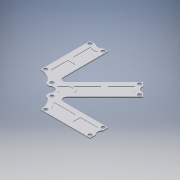
# Autodesk Inventor part: SolarFolds_Sketch
Saved by Autodesk Inventor 2016 (Build 200138000, 138)
## iProperties
Created: 2015-03-28
Part Number: SolarFolds_Sketch
Material: Generic
Document SubType Name: Modeling
Designer: Erin
Density: 1 g/cm^3
Appearance: Default
Author: Erin
Autodesk Inventor part; units mm, degrees
ref_plane "YZ Plane" through (0, 0, 0) normal (1, 0, 0) x (0, 1, 0)
ref_plane "XZ Plane" through (0, 0, 0) normal (0, 1, 0) x (-1, 0, 0)
sketch "Sketch1" plane through (0, 0, 0) normal (0, 0, 1) x (1, 0, 0)
  line L0 (-41.5, 58) -> (41.5, 58)
  line L1 (41.5, 58) -> (41.5, 158)
  line L2 (41.5, 158) -> (-41.5, 158)
  line L3 (-41.5, 158) -> (-41.5, 58)
  line L4 (58, 41.5) -> (158, 41.5)
  line L5 (158, 41.5) -> (158, -41.5)
  line L6 (158, -41.5) -> (58, -41.5)
  line L7 (58, -41.5) -> (58, 41.5)
  line L8 (-131.1952, 0) -> (204.4844, 0) construction
  line L9 (-48, 48) -> (48, 48)
  line L10 (48, 48) -> (48, -48)
  line L11 (48, -48) -> (-48, -48)
  line L12 (-48, -48) -> (-48, 48)
  line L13 (0, 180.9439) -> (0, -136.3054) construction
  point P0 (0, 0)
  point P1 (-48, 0)
  point P2 (0, 48)
  point P3 (0, 58)
  point P4 (58, 0)
  dimension "d0" = 83
  dimension "d1" = 100
  dimension "d2" = 100
  dimension "d3" = 83
  dimension "d5" = 96
  dimension "d6" = 96
  dimension "d7" = 10
  dimension "d8" = 10
  constraints: 28 end point, 7 parallel, 4 horizontal, 4 midpoint, 4 perpendicular, 2 horizontal alignment, 2 vertical alignment, 1 vertical
  measures "d0" distance of L2.end L1.end
  measures "d1" distance of L1.end L0.end
  measures "d2" distance of L5.end L6.end
  measures "d3" distance of L4.end L5.end
  measures "d5" distance of L9.start L9.end
  measures "d6" distance of L11.end L9.start
  measures "d7" distance between parallel lines of L9 L0
  measures "d8" distance between parallel lines of L7 L10
sketch "Sketch2" plane through (0, 0, 0) normal (0, 0, 1) x (1, 0, 0)
  line L0 (41.5, 158) -> (-41.5, 158) projected
  line L1 (41.5, 58) -> (41.5, 158) projected
  line L2 (-48, 48) -> (48, 48) projected
  line L3 (48, 48) -> (48, -48) projected
  line L4 (58, -41.5) -> (58, 41.5) projected
  line L5 (58, 41.5) -> (158, 41.5) projected
  line L6 (-41.5, 58) -> (41.5, 58) projected
  line L7 (158, 41.5) -> (158, -41.5) projected
  line L8 (48, 48) -> (136.7868, 136.7868) construction
  line L9 (35.5, 78) -> (57.5, 78)
  line L10 (57.5, 78) -> (57.5, 138)
  line L11 (57.5, 138) -> (35.5, 138)
  line L12 (35.5, 138) -> (35.5, 78)
  line L13 (41.5, 108) -> (-41.5, 108) construction
  line L14 (108, 41.5) -> (108, -41.5) construction
  line L15 (41.5, 158) -> (220.1006, 158) construction
  line L16 (158, 41.5) -> (158, 206.0131) construction
  line L17 (115.5736, 158) -> (158, 115.5736) construction
  line L18 (41.5, 138) -> (41.5, 78) construction
  line L19 (51.5, 138) -> (51.5, 78) construction
  line L20 (46.5, 138) -> (46.5, 78) construction
  line L21 (51.5, 158) -> (51.5, 70.6421)
  line L22 (60.0355, 67.1066) -> (133.2513, 140.3223)
  arc A0 (51.5, 158) -> (133.2513, 140.3223) centre (109.2071, 226.9991) ccw
  line L23 (68.9045, 84.4609) -> (84.4609, 68.9045)
  line L24 (84.4609, 68.9045) -> (126.8873, 111.331)
  line L25 (126.8873, 111.331) -> (111.331, 126.8873)
  line L26 (111.331, 126.8873) -> (68.9045, 84.4609)
  line L27 (80.2183, 73.1472) -> (122.6447, 115.5736) construction
  line L28 (105.6741, 90.1177) -> (90.1177, 105.6741) construction
  line L29 (73.1472, 80.2183) -> (115.5736, 122.6447) construction
  line L30 (76.6827, 76.6827) -> (119.1091, 119.1091) construction
  circle A1 centre (73.1472, 84.4609) radius 2.25
  circle A2 centre (111.331, 122.6447) radius 2.25
  circle A3 centre (84.4609, 73.1472) radius 2.25
  circle A4 centre (122.6447, 111.331) radius 2.25
  circle A5 centre (38.5, 135) radius 2.25
  circle A6 centre (38.5, 81) radius 2.25
  circle A7 centre (54.5, 135) radius 2.25
  circle A8 centre (54.5, 81) radius 2.25
  arc A9 (51.5, 70.6421) -> (60.0355, 67.1066) centre (56.5, 70.6421) ccw
  point P0 (0, 0)
  point P1 (158, 158)
  dimension "d23" = 30
  dimension "d25" = 45
  dimension "d30" = 10
  dimension "d37" = 10
  dimension "d38" = 60
  dimension "d39" = 4.5
  dimension "d40" = 3
  dimension "d42" = 4.5
  dimension "d43" = 3
  dimension "d46" = 60
  dimension "d47" = 30
  dimension "d48" = 4.5
  dimension "d49" = 3
  dimension "d50" = 3
  dimension "d51" = 4.5
  dimension "d52" = 3
  dimension "d53" = 3
  dimension "d54" = 5
  dimension "d55" = 25
  dimension "d57" = 3
  dimension "d58" = 3
  dimension "d59" = 3
  dimension "d60" = 3
  constraints: 46 end point, 15 perpendicular, 14 point on line, 10 centre point, 9 midpoint, 5 collinear, 4 point on circle, 4 symmetric about line, 3 parallel, 2 tangent, 1 horizontal, 4 other
  measures "d23" distance from line of point (158, 158) L17
  measures "d25" angle of L16 L17
  measures "d30" distance between parallel lines of L18 L19
  measures "d37" distance between parallel lines of L27 L29
  measures "d38" distance of L23.end L24.end
  measures "d39" diameter of A1
  measures "d40" distance from line of A1.centre L26
  measures "d42" diameter of A2
  measures "d43" distance from line of A2.centre L26
  measures "d46" distance of L9.end L10.end
  measures "d47" distance between parallel lines of L13 L11
  measures "d48" diameter of A5
  measures "d49" distance from line of A5.centre L11
  measures "d50" distance from line of A5.centre L12
  measures "d51" diameter of A6
  measures "d52" distance from line of A6.centre L9
  measures "d53" distance from line of A6.centre L12
  measures "d54" radius of A9
  measures "d55" distance between parallel lines of L17 L25
  measures "d57" distance from line of A5.centre L1
  measures "d58" distance from line of A7.centre L21
  measures "d59" distance from line of A4.centre L27
  measures "d60" distance from line of A2.centre L22
sketch "Sketch6" plane through (0, 0, 0) normal (0, 0, 1) x (1, 0, 0)
  line L0 (57.5, 138) -> (35.5, 138) projected
  line L1 (35.5, 138) -> (35.5, 78) projected
  line L2 (35.5, 78) -> (57.5, 78) projected
  circle A0 centre (38.5, 81) radius 2.25 projected
  circle A1 centre (38.5, 135) radius 2.25 projected
  circle A2 centre (54.5, 135) radius 2.25 projected
  line L3 (111.331, 126.8873) -> (68.9045, 84.4609) projected
  circle A3 centre (111.331, 122.6447) radius 2.25 projected
  line L4 (126.8873, 111.331) -> (111.331, 126.8873) projected
  line L5 (84.4609, 68.9045) -> (126.8873, 111.331) projected
  line L6 (68.9045, 84.4609) -> (84.4609, 68.9045) projected
  line L7 (60.0355, 67.1066) -> (133.2513, 140.3223) projected
  arc A4 (51.5, 70.6421) -> (60.0355, 67.1066) centre (56.5, 70.6421) ccw projected
  line L8 (51.5, 158) -> (51.5, 70.6421) projected
  arc A5 (51.5, 158) -> (133.2513, 140.3223) centre (109.2071, 226.9991) ccw projected
  line L9 (119.1091, 119.1091) -> (76.6827, 76.6827) construction
  circle A6 centre (38.5, 135) radius 2.25
  circle A7 centre (38.5, 81) radius 2.25
  circle A8 centre (54.5, 135) radius 2.25
  circle A9 centre (111.331, 122.6447) radius 2.25
  circle A10 centre (56.5, 70.6421) radius 2.25
  line L10 (57.5, 138) -> (51.5, 138)
  line L11 (35.5, 138) -> (35.5, 78)
  line L12 (57.5, 138) -> (57.5, 83.3339)
  line L13 (111.331, 126.8873) -> (64.3853, 79.9416)
  line L14 (111.331, 126.8873) -> (115.5736, 122.6447)
  line L15 (126.8873, 111.331) -> (84.4609, 68.9045)
  arc A11 (51.5, 70.6421) -> (60.0355, 67.1066) centre (56.5, 70.6421) ccw
  arc A12 (51.5, 70.6421) -> (35.5, 78) centre (33.8506, 53.3381) ccw
  arc A13 (42.2688, 138) -> (51.5, 138) centre (46.8844, 142.3576) ccw
  line L16 (42.2688, 138) -> (35.5, 138)
  arc A14 (115.5736, 122.6447) -> (123.8972, 114.3211) centre (123.1928, 121.9402) ccw
  line L17 (123.8972, 114.3211) -> (126.8873, 111.331)
  arc A15 (57.5, 83.3339) -> (64.3853, 79.9416) centre (61.7783, 83.3339) ccw
  arc A16 (66.0227, 66.0227) -> (60.0355, 67.1066) centre (61.5732, 58.5223) ccw
  line L18 (66.0227, 66.0227) -> (76.6827, 76.6827)
  line L19 (76.6827, 76.6827) -> (84.4609, 68.9045)
  point P0 (0, 0)
  point P1 (69.6117, 76.6827)
  dimension "d99" = 4.5
  constraints: 22 end point, 12 point on circle, 11 centre point, 5 coincident, 4 collinear, 4 concentric, 4 point on line, 3 perpendicular, 3 tangent, 2 horizontal, 2 midpoint, 1 vertical
  measures "d99" diameter of A10
extrude "Extrusion13" add sketch "Sketch6" along normal blind 0.6 contours L12 A15 L13 L6 L7 A4 L8 L0 | L8 L2 L1 L0 A13 | L8 A12 L2 | L3 L4 L7 L6 | A14 L4 L5 L6 L7 | L7 L6 L18 A16 | A2 | A3 | A10
ref_plane "Work Plane5" through (119.1091, 119.1091, 0) normal (-0.7071, 0.7071, 0) x (-0.7071, -0.7071, 0)
mirror "Mirror3" about plane through (119.1091, 119.1091, 0) normal (-0.7071, 0.7071, 0) of "Extrusion13"
extrude "Extrusion14" cut sketch "Sketch6" along normal blind 0.6 contours A3
mirror "Mirror4" about plane through (119.1091, 119.1091, 0) normal (-0.7071, 0.7071, 0) of "Extrusion14"
sketch "Sketch8" plane through (0, 0, 0.6) normal (0, 0, 1) x (1, 0, 0)
  line L0 (57.5, 138) -> (51.5, 138) projected
  arc A0 (51.5, 70.6421) -> (60.0355, 67.1066) centre (56.5, 70.6421) ccw projected
  line L1 (57.5, 138) -> (51.5, 138)
  line L2 (51.5, 138) -> (51.5, 70.6421)
  line L3 (51.5, 70.6421) -> (57.5, 70.6421)
  line L4 (57.5, 70.6421) -> (57.5, 138)
  line L5 (35.5, 138) -> (35.5, 78) projected
  line L6 (35.5, 138) -> (42.2688, 138)
  line L7 (42.2688, 138) -> (42.2688, 76.5774)
  line L8 (42.2688, 76.5774) -> (35.5, 76.5774)
  line L9 (35.5, 76.5774) -> (35.5, 138)
  arc A1 (51.5, 70.6421) -> (35.5, 78) centre (33.8506, 53.3381) ccw projected
  arc A2 (42.2688, 131.917) -> (51.5, 131.7579) centre (47.0049, 138.8311) ccw
  line L10 (35.5, 107.2887) -> (57.5, 107.2887) construction
  line L11 (57.5, 83.3339) -> (57.5, 138) projected
  line L12 (35.5, 110.2887) -> (57.5, 110.2887)
  line L13 (57.5, 110.2887) -> (57.5, 104.2887)
  line L14 (57.5, 104.2887) -> (35.5, 104.2887)
  line L15 (35.5, 104.2887) -> (35.5, 110.2887)
  line L16 (111.331, 126.8873) -> (115.5736, 122.6447)
  line L17 (115.5736, 122.6447) -> (60.0355, 67.1066)
  line L18 (60.0355, 67.1066) -> (55.7929, 71.3492)
  line L19 (55.7929, 71.3492) -> (111.331, 126.8873)
  line L20 (64.3853, 79.9416) -> (111.331, 126.8873) projected
  line L21 (64.3853, 79.9416) -> (111.331, 126.8873) projected
  line L22 (87.8581, 103.4145) -> (103.4145, 87.8581) construction
  line L23 (79.9416, 64.3853) -> (126.8873, 111.331) projected
  line L24 (89.9794, 105.5358) -> (105.5358, 89.9794)
  line L25 (105.5358, 89.9794) -> (101.2931, 85.7368)
  line L26 (101.2931, 85.7368) -> (85.7368, 101.2931)
  line L27 (85.7368, 101.2931) -> (89.9794, 105.5358)
  arc A3 (51.5, 70.6421) -> (60.0355, 67.1066) centre (56.5, 70.6421) ccw
  arc A4 (57.5, 83.3339) -> (64.3853, 79.9416) centre (61.7783, 83.3339) ccw projected
  arc A5 (57.5, 83.3339) -> (64.3853, 79.9416) centre (61.7783, 83.3339) ccw
  arc A6 (76.6827, 76.6827) -> (69.6117, 76.6827) centre (73.1472, 72.5977) ccw
  line L28 (76.6827, 76.6827) -> (78.804, 78.804)
  arc A7 (78.804, 78.804) -> (73.1472, 80.2183) centre (74.8151, 74.869) ccw
  line L29 (42.2688, 131.917) -> (42.2688, 138)
  line L30 (51.5, 131.7579) -> (51.5, 138)
  line L31 (73.1472, 80.2183) -> (69.6117, 76.6827)
  line L32 (126.8873, 111.331) -> (122.6447, 115.5736) projected
  arc A8 (117.1923, 117.1923) -> (122.6447, 115.5736) centre (121.9402, 123.1928) ccw projected
  arc A9 (115.5736, 122.6447) -> (122.6447, 115.5736) centre (121.4114, 121.4114) ccw
  arc A10 (110.6174, 117.6885) -> (113.3377, 113.3377) centre (121.4114, 121.4114) ccw
  arc A11 (115.5736, 122.6447) -> (117.1923, 117.1923) centre (123.1928, 121.9402) ccw projected
  line L33 (111.331, 126.8873) -> (115.5736, 122.6447) projected
  line L34 (115.5736, 122.6447) -> (110.6174, 117.6885)
  arc A12 (51.5, 77.7274) -> (35.5, 84.6602) centre (34.6745, 60.8256) ccw
  line L35 (35.5, 85.7368) -> (35.5, 78)
  line L36 (51.5, 78.804) -> (51.5, 70.6421)
  arc A13 (51.5, 70.6421) -> (35.5, 78) centre (33.8506, 53.3381) ccw
  arc A14 (42.2688, 138) -> (51.5, 138) centre (46.8844, 142.3576) ccw projected
  line L37 (42.2688, 138) -> (35.5, 138) projected
  arc A15 (42.2688, 138) -> (51.5, 138) centre (46.8844, 142.3576) ccw
  line L38 (117.1923, 117.1923) -> (113.3377, 113.3377)
  arc A16 (68.3773, 68.3773) -> (63.1267, 70.1978) centre (62.8115, 60.8068) ccw
  arc A17 (66.0227, 66.0227) -> (60.0355, 67.1066) centre (61.5732, 58.5223) ccw projected
  line L39 (68.3773, 68.3773) -> (66.0227, 66.0227)
  line L40 (57.5, 138) -> (57.5, 83.3339) projected
  line L41 (57.5, 83.3339) -> (57.5, 73.0563)
  line L42 (57.5, 73.0563) -> (64.3853, 79.9416)
  point P0 (0, 0)
  point P1 (35.5, 107.2887)
  dimension "d114" = 6
  dimension "d117" = 3
  constraints: 66 end point, 24 point on circle, 12 point on line, 11 centre point, 11 parallel, 7 collinear, 6 perpendicular, 4 midpoint, 3 concentric, 3 horizontal, 2 coincident, 1 vertical
  measures "d114" distance of L12.end L13.end
  measures "d117" distance of L28.start L28.end
extrude "Extrusion15" add sketch "Sketch8" along normal blind 0.6 contours L4 L12 L2 L0 | L2 A2 L7 A14 | L4 L14 L2 L12 | L7 L12 L5 L6 | L4 L19 L18 L3 L2 L14 | L2 L14 L7 L12 | A4 L19 L4 | L7 L14 L5 L12 | L19 L26 L17 L18 L3 L4 | L4 L3 L18 L19 | L7 A12 L5 L14 | L19 L24 L17 L26 | L2 A1 L7 A12 | L7 A1 L5 A12 | L18 A0 L3 | L19 L16 L17 L24 | L17 L24 L23 L26 | L17 A16 L39 A17 | A7 L28 A6 L17 | A9 L38 A10 L17 | A11 A9
extrude "Extrusion16" cut sketch "Sketch6" along normal blind 3 contours A0 | A1 | A2 | A3 | A10
mirror "Mirror5" about plane through (119.1091, 119.1091, 0) normal (-0.7071, 0.7071, 0) of "Extrusion15", "Extrusion16"
body "Solid2"
